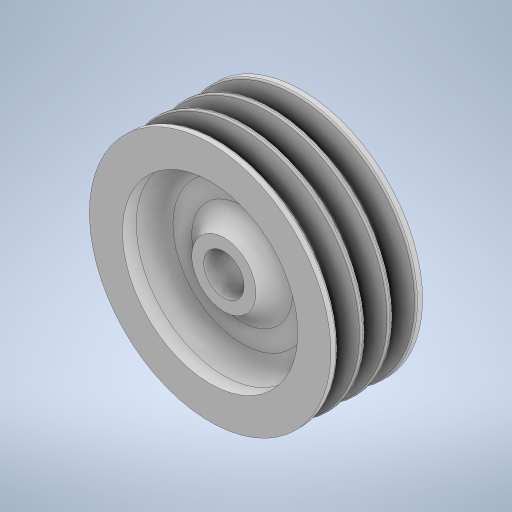
# Autodesk Inventor part: S3-SPS-REMENICE-0
Saved by Autodesk Inventor 2024 (Build 280153000, 153)
## iProperties
Created: 2023-12-19
Part Number: S3-SPS-REMENICE-0
Material: Všeobecné
Document SubType Name: Modeling
Designer: S21Suk
Density: 1 g/cm^3
Appearance: Výchozí
MASSSFP: 400 g
SFP: 4HR
Author: S21Suk
Autodesk Inventor part; units mm, degrees
ref_plane "YZ Plane" through (0, 0, 0) normal (1, 0, 0) x (0, 1, 0)
ref_plane "XZ Plane" through (0, 0, 0) normal (0, 1, 0) x (-1, 0, 0)
ref_plane "XY Plane" through (0, 0, 0) normal (0, 0, 1) x (1, 0, 0)
sketch "Náčrt2" plane through (0, 0, 0) normal (1, 0, 0) x (0, 1, 0)
  line L0 (0, 0) -> (0, -50)
  line L1 (0, 0) -> (62.5, 0)
  line L2 (62.5, 0) -> (65.8, 0)
  line L3 (65.8, -50) -> (0, -50)
  line L4 (62.5, 0) -> (53.8, 0)
  line L5 (17.5, 0) -> (17.5, -50)
  line L6 (62.5, 0) -> (62.5, -50) construction
  line L7 (53.8, 0) -> (53.8, -50)
  line L8 (65.8, 0) -> (65.8, -50)
  line L9 (65.8, -17.5) -> (17.5, -17.5)
  line L10 (65.8, -32.5) -> (17.5, -32.5)
  line L11 (65.8, -10) -> (53.8, -10)
  line L12 (65.8, -10) -> (65.8, -16.5) construction
  line L13 (65.8, -16.5) -> (53.8, -12.601)
  line L14 (65.8, -3.5) -> (53.8, -7.399)
  line L15 (65.8, -18.5) -> (53.8, -22.399)
  line L16 (65.8, -31.5) -> (53.8, -27.601)
  line L17 (65.8, -46.5) -> (53.8, -42.601)
  line L18 (65.8, -33.5) -> (53.8, -37.399)
  line L19 (11, -50) -> (11, 0)
  line L20 (65.8, -25) -> (0, -25)
  line L21 (17.5, -7.5) -> (0, -7.5)
  line L22 (17.5, -42.5) -> (0, -42.5)
  line L23 (17.5, -22) -> (53.8, -22)
  line L24 (17.5, -28) -> (53.8, -28)
  line L25 (47.8, 0) -> (47.8, -50)
  point P0 (17.5, -25)
  point P1 (11, -7.5)
  point P2 (11, -42.5)
  point P3 (47.8, -32.5)
  point P4 (47.8, -17.5)
  dimension "d2" = 50
  dimension "d3" = 62.5
  dimension "d4" = 3.3
  dimension "d5" = 50
  dimension "d10" = 17.5
  dimension "d16" = 8.7
  dimension "d27" = 17.5
  dimension "d28" = 15
  dimension "d30" = 10
  dimension "d31" = 6.5
  dimension "d32" = 18
  dimension "d34" = 11
  dimension "d35" = 17.5
  dimension "d36" = 3
  dimension "d37" = 6
  constraints: 52 end point, 21 point on line, 14 symmetric about line, 10 perpendicular, 3 midpoint, 2 horizontal, 2 vertical
  measures "d2" distance of L0.start L0.end
  measures "d3" distance of L0.start L1.end
  measures "d4" distance of L1.end L2.end
  measures "d5" distance of L2.end L3.start
  measures "d10" distance from line of L5 L0.start
  measures "d16" distance between parallel lines of L7 L6
  measures "d27" distance of L9.start L2.end
  measures "d28" distance of L10.start L9.start
  measures "d30" distance of L11.start L2.end
  measures "d31" distance of L11.start L12.end
  measures "d32" angle of L13 L11
  measures "d34" distance from line of L0.end L19
  measures "d35" distance of L20.end L21.end
  measures "d36" distance of point (17.5, -25) L23.start
  measures "d37" distance of L4.end L25.start
revolve "Rotace1" add sketch "Náčrt2" angle 360 about axis through (0, 0, 0) along (0, 0, -1) contours L21 L5 L20 L19 | L20 L5 L22 L19 | L1 L7 L9 L25 | L20 L25 L24 L5 | L5 L23 L25 L20 | L9 L25 L23 L5 | L1 L2 L8 L14 L7 | L9 L7 L23 L25 | L24 L25 L10 L5 | L25 L23 L7 L20 | L20 L7 L24 L25 | L9 L8 L15 L7 | L7 L13 L8 L9 | L24 L7 L10 L25 | L25 L10 L7 L3 | L7 L16 L8 L10 | L7 L17 L8 L3 | L10 L8 L18 L7
fillet "Zaoblení2" radius 1 6 edges at (0, -65.8, -46.5) (0, -65.8, -33.5) (0, -65.8, -31.5) (0, -65.8, -16.5) (0, -65.8, -18.5) (0, -65.8, -3.5)
fillet "Zaoblení3" radius 10 4 edges at (0, -17.5, -17.5) (0, -47.8, -17.5) (0, -17.5, -32.5) (0, -47.8, -32.5)
